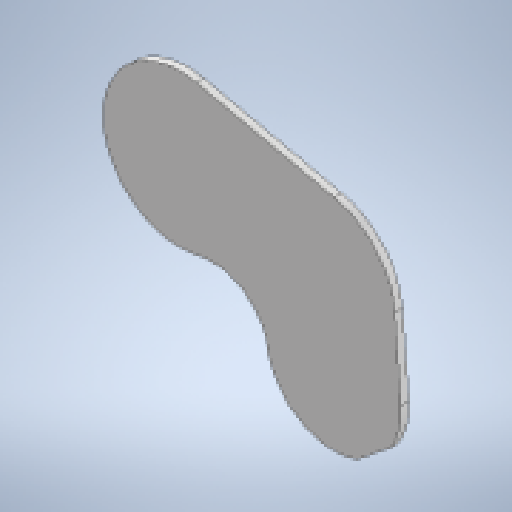
# Autodesk Inventor part: Peça2
Saved by Autodesk Inventor 2025.2 (Build 292293000, 293)
## iProperties
Created: 2025-06-03
Part Number: Peça2
Material: Genérico
Document SubType Name: Modeling
Designer: Gustavo Sousa
Density: 1 g/cm^3
Appearance: Branco
Author: Gustavo Sousa
Autodesk Inventor part; units mm, degrees
sketch "Esboço1" plane through (0, 0, 0) normal (0, 0, 1) x (1, 0, 0)
  arc A0 (3.678, 19.15) -> (4.657, -18.9358) centre (0, 0) ccw
  line L0 (3.678, 19.15) -> (39.7998, 12.2124)
  line L1 (57.7995, -7.9297) -> (59.2705, -26.8636)
  arc A1 (56.1556, -38.4578) -> (59.2705, -26.8636) centre (41.3246, -28.2578) ccw
  arc A2 (24.8291, -31.7542) -> (47.6703, -45.4578) centre (42.4793, -28.2226) ccw
  arc A3 (57.7995, -7.9297) -> (39.7998, 12.2124) centre (35.6, -9.6544) ccw
  line L2 (56.1556, -38.4578) -> (47.6703, -45.4578)
  arc A4 (24.8291, -31.7542) -> (4.657, -18.9358) centre (8.6077, -35) ccw
  point P0 (17.4802, -21.0376)
  point P1 (51.913, -41.9578)
  point P2 (33.2189, -43.6578)
  point P3 (58.7081, -32.928)
  point P4 (58.535, -17.3966)
  dimension "d6" = 19.5
  dimension "d30" = 8.6077
  dimension "d34" = 35
  dimension "d35" = 51
  dimension "d36" = 13.7
  dimension "d37" = 17.2
  dimension "d38" = 15.4
  dimension "d39" = 18
  dimension "d40" = 11
  dimension "d41" = 18
  dimension "d42" = 22.935
  dimension "d43" = 35.6
  dimension "d44" = 19.15
  constraints: 13 point on circle, 6 end point, 6 tangent, 5 centre point, 2 midpoint, 1 coincident
  measures "d6" radius of A0
  measures "d30" horizontal distance of A4.centre point (0, 0)
  measures "d34" vertical distance of point (0, 0) A4.centre
  measures "d35" distance of point (0, 0) A2.centre
  measures "d36" vertical distance of A1.centre point (51.913, -41.958)
  measures "d37" vertical distance of A1.centre L2.end
  measures "d38" vertical distance of A1.centre point (33.219, -43.658)
  measures "d39" radius of A2
  measures "d40" distance of L2.start L2.end
  measures "d41" radius of A1
  measures "d42" horizontal distance of A3.centre point (58.535, -17.397)
  measures "d43" horizontal distance of A0.centre A3.centre
  measures "d44" vertical distance of point (0, 0) L0.start
extrude "Extrusão1" add sketch "Esboço1" along normal mid plane 2
